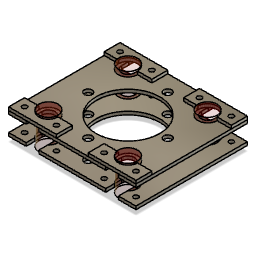
RT 60K thermal separator v4 (Autodesk Fusion 360 design; units mm, degrees)
Autodesk Fusion 360 part; units mm, degrees
note: some values were not read from the file. Chosen so that the rebuilt part matches the saved one: a direction; which face or edge a step refers to. Set by a fixed rule: which sketch regions a step uses.
sketch "Sketch1" plane through (0, 0, 0) normal (0, 1, 0) x (1, 0, 0)
  line L0 (-40, 35) -> (40, 35)
  line L1 (40, 35) -> (40, -35)
  line L2 (40, -35) -> (-40, -35)
  line L3 (-40, -35) -> (-40, 35)
  line L4 (-29, 35) -> (-29, 25)
  arc A0 (-29, 25) -> (-21, 25) centre (-25, 25) ccw
  line L5 (-21, 25) -> (-21, 35)
  line L6 (1.75, 0) -> (22.5, 0) construction
  line L7 (0, -1.75) -> (0, -22.5) construction
  line L8 (29, 35) -> (29, 25)
  arc A1 (21, 25) -> (29, 25) centre (25, 25) ccw
  line L9 (21, 25) -> (21, 35)
  line L10 (-40, 0) -> (40, 0) construction
  line L11 (-29, -35) -> (-29, -25)
  arc A2 (-21, -25) -> (-29, -25) centre (-25, -25) ccw
  line L12 (-21, -25) -> (-21, -35)
  line L13 (29, -35) -> (29, -25)
  arc A3 (29, -25) -> (21, -25) centre (25, -25) ccw
  line L14 (21, -25) -> (21, -35)
  circle A4 centre (-25, 25) radius 4
  circle A5 centre (-25, 25) radius 6
  line L15 (-25, 25) -> (-25, 35) construction
  line L16 (-40, 25) -> (-10, 25)
  line L17 (-10, 25) -> (-10, 35)
  circle A6 centre (0, 0) radius 20
  point P0 (-35, 30)
  point P1 (-15, 30)
  point P2 (15, 30)
  point P3 (35, 30)
  point P4 (-35, -30)
  point P5 (-15, -30)
  point P6 (15, -30)
  point P7 (35, -30)
  point P8 (0, 25)
  point P9 (-25, 0)
  point P10 (25, 0)
  point P11 (0, -25)
  dimension "d2" = 8
  dimension "d3" = 10
  dimension "d7" = 12
  dimension "d11" = 20
  dimension "d13" = 50
  dimension "d14" = 50
  dimension "d15" = 15
  dimension "d16" = 50
  dimension "d17" = 50
  dimension "d53" = 5
  dimension "d54" = 40
  constraint horizontal L0
  constraint vertical L1
  constraint horizontal L2
  constraint vertical L3
  constraint coincident L0 L4.start
  constraint perpendicular L0 L4
  constraint tangent L4 A0
  constraint coincident L0 L5.end
  constraint tangent A0 L5
  constraint perpendicular L0 L5
  constraint symmetric L1 L3 L7
  constraint symmetric L4.start L7 L8.start
  constraint symmetric L4.end L7 L8.end
  constraint symmetric A0.end L7 A1.start
  constraint symmetric A0 L7 A1
  constraint symmetric L5.end L7 L9.end
  constraint midpoint L3 L10.start
  constraint midpoint L1 L10.end
  constraint symmetric L4.start L10 L11.start
  constraint symmetric L4.end L10 L11.end
  constraint symmetric A0.end L10 A2.start
  constraint symmetric A0 L10 A2
  constraint symmetric L5.end L10 L12.end
  constraint symmetric L8.end L10 L13.end
  constraint symmetric A1.start L10 A3.end
  constraint symmetric L8.start L10 L13.start
  constraint symmetric A1 L10 A3
  constraint symmetric L9.end L10 L14.end
  constraint concentric A0 A4
  constraint coincident L4.end A4
  constraint concentric A4 A5
  constraint coincident A6.centre L10
  constraint horizontal P0 P1
  constraint coincident A0.centre A4.centre
  constraint coincident L0 L15.end
  constraint perpendicular L0 L15
  constraint symmetric P0 P1 L15
  constraint perpendicular L15 L16
  constraint coincident L0 L17.end
  constraint perpendicular L0 L17
  constraint coincident A0.centre L16
  constraint symmetric L7 P0 P3
  constraint symmetric L7 P1 P2
  constraint symmetric L10 P0 P4
  constraint symmetric L10 P1 P5
  constraint symmetric L10 P2 P6
  constraint symmetric L10 P3 P7
  constraint coincident L10 P9
  constraint coincident L10 P10
  constraint coincident L7 P11
  constraint coincident L7 P8
  constraint symmetric L10 P8 P11
  constraint symmetric L7 P9 P10
  constraint coincident L3 L16.start
  constraint coincident A6.centre origin
  measures "d2" distance of L4 L5
  measures "d3" distance of L0 A0.centre
  measures "d7" diameter of A5
  measures "d11" distance of P0 P1
  measures "d13" distance of A2.centre A0.centre
  measures "d14" distance of A1.centre A0.centre
  measures "d15" distance of L3 A0.centre
  measures "d16" distance of P8 P11
  measures "d17" distance of P9 P10
  measures "d53" distance of L0 P0
  measures "d54" diameter of A6
extrude "Extrude1" add sketch "Sketch1" along normal blind 2 from surface at 5 contours L0 L3 L4 A5 L16 | L0 L1 L2 L3 L8 A1 L9 L11 A2 L12 L13 A3 L14 A5 L16 L17 | L0 L5 A5 L16 L17 | L4 A5 L16 | A0 A4 A5 L16 | L5 A5 L16 makes body 1
extrude "Extrude3" add sketch "Sketch1" along normal mid plane 10 separate body contours L4 L5 A4 A5 | L4 A5 L16 | A0 A4 A5 L16 | L5 A5 L16 | A0 A4 L16 | A4 L16 makes body 2
extrude "Extrude4" add sketch "Sketch1" along normal mid plane 14 contours L4 L5 A4 A5 | A0 A4 L16 | A4 L16 bodies 2
extrude "Extrude5" add sketch "Sketch1" along normal blind 3 from surface at 7 contours L4 L5 A4 A5 | L4 A5 L16 | A0 A4 A5 L16 | L5 A5 L16 | A0 A4 L16 | A4 L16 bodies 2
mirror "Mirror1" about plane through (0, 0, 0) normal (0, 1, 0) of "Extrude5"
extrude "Extrude6" add sketch "Sketch1" along normal blind 2 from surface at 7 separate body contours L0 L3 L4 A5 L16 | L0 L4 L5 A5 | L0 L5 A5 L16 L17 makes body 3
hole "Hole1" at (0, 0, 25) at (-25, 0, 0) at (0, 0, -25) at (25, 0, 0) direction (0, 1, 0) diameter 5 end through all bodies 1
hole "Hole3" at (-35, 0, -30) at (-15, 0, -30) at (15, 0, -30) at (35, 0, -30) at (35, 0, 30) at (15, 0, 30) at (-15, 0, 30) at (-35, 0, 30) direction (0, 1, 0) diameter 3 end through all bodies 3 1
copy_body "Body->Comp1" bodies 1 removing the originals makes body 4 in component "Ti Baseplate"
copy_body "Body->Comp2" bodies 2 removing the originals makes body 5 in component "Vespel spacer"
copy_body "Body->Comp3" bodies 3 removing the originals makes body 6 in component "Ti clamp"
mirror "MirrorComponent1" about plane through (0, 0, 0) normal (0, 0, 1) of bodies 5 makes body 7 in component "Vespel spacer(Mirror)"
mirror "MirrorComponent1'" about plane through (0, 0, 0) normal (0, 0, 1) of bodies 6 makes body 8 in component "Ti clamp(Mirror)"
mirror "MirrorComponent2" about plane through (0, 0, 0) normal (0, 0, 1) of bodies 5 makes body 9 in component "Vespel spacer(Mirror) (1)"
mirror "MirrorComponent2'" about plane through (0, 0, 0) normal (0, 0, 1) of bodies 6 makes body 10 in component "Ti clamp(Mirror) (1)"
mirror "MirrorComponent2''" about plane through (0, 0, 0) normal (0, 0, 1) of bodies 8 makes body 11 in component "Ti clamp(Mirror)(Mirror)"
mirror "MirrorComponent2'''" about plane through (0, 0, 0) normal (0, 0, 1) of bodies 7 makes body 12 in component "Vespel spacer(Mirror)(Mirror)"
mirror "MirrorComponent3" about plane through (0, 0, 0) normal (0, 0, 1) of bodies 4 makes body 13 in component "Ti Baseplate(Mirror)"
component "Ti Baseplate" placed x (1, 0, 0) y (0, 1, 0) z (0, 0, 1) at (0, 0, 0)
component "Vespel spacer" placed x (1, 0, 0) y (0, 1, 0) z (0, 0, 1) at (0, 0, 0)
component "Ti clamp" placed x (1, 0, 0) y (0, 1, 0) z (0, 0, 1) at (0, 0, 0)
component "Vespel spacer(Mirror)" placed x (1, 0, 0) y (0, 1, 0) z (0, 0, 1) at (0, 0, 0)
component "Ti clamp(Mirror)" placed x (1, 0, 0) y (0, 1, 0) z (0, 0, 1) at (0, 0, 0)
component "Vespel spacer(Mirror) (1)" placed x (-1, 0, 0) y (0, 1, 0) z (0, 0, -1) at (0, 0, 0)
component "Ti clamp(Mirror) (1)" placed x (-1, 0, 0) y (0, 1, 0) z (0, 0, -1) at (0, 0, 0)
component "Vespel spacer(Mirror)(Mirror)" placed x (-1, 0, 0) y (0, 1, 0) z (0, 0, -1) at (0, 0, 0)
component "Ti clamp(Mirror)(Mirror)" placed x (-1, 0, 0) y (0, 1, 0) z (0, 0, -1) at (0, 0, 0)
component "Ti Baseplate(Mirror)" placed x (1, 0, 0) y (0, -1, 0) z (0, 0, -1) at (0, 0, 0)
equation "d13 = mainDim"
equation "d14 = mainDim"
equation "d16 = mainDim"
equation "d17 = mainDim"
equation "mainDim = 50 mm"
equation "plateDistance = 10 mm"
equation "d20 = plateDistance / 2"
equation "d21 = plateThickness"
equation "plateThickness = 2 mm"
equation "d27 = plateDistance"
named bodies: "Ti Baseplate", "Vespel spacer", "Ti clamp"
